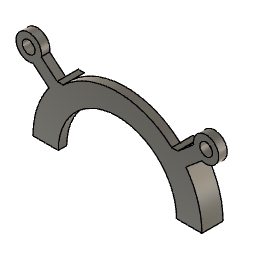
v2 - Timer - Assembly (Autodesk Fusion 360 archive; units mm, degrees)
design "v2 - Timer - Led ring insert"
Autodesk Fusion 360 part; units mm, degrees
note: some values were not read from the file. Chosen so that the rebuilt part matches the saved one: which bodies a step acts on; which face or edge a step refers to. Set by a fixed rule: which sketch regions a step uses.
sketch "Sketch1" plane through (0, 0, 0) normal (0, 1, 0) x (1, 0, 0)
  line L0 (0, 0) -> (50, 0)
  line L1 (50, 0) -> (50, -38.7)
  line L2 (50, -38.7) -> (0, -38.7)
  line L3 (0, -38.7) -> (0, 0)
  line L4 (0, -38.7) -> (50, -38.7)
  line L5 (50, -38.7) -> (50, -23.7)
  line L6 (50, -23.7) -> (0, -23.7)
  line L7 (0, -23.7) -> (0, -38.7)
  circle A0 centre (46, -17.7) radius 1.5
  circle A1 centre (4, -17.7) radius 1.5
  circle A2 centre (25, 0) radius 20
  circle A3 centre (25, 0) radius 1.5
  line L8 (3.0333, -16.5531) -> (24.0333, 1.1469)
  line L9 (4.9667, -18.8469) -> (25.9667, -1.1469)
  line L10 (45.0333, -18.8469) -> (24.0333, -1.1469)
  line L11 (46.9667, -16.5531) -> (25.9667, 1.1469)
  circle A4 centre (4, -17.7) radius 3
  circle A5 centre (46, -17.7) radius 3
  circle A6 centre (25, 0) radius 14
  circle A7 centre (25, 0) radius 19
  line L12 (39.2828, -14.0001) -> (10.7172, -14.0001)
  dimension "d1" = 50
  dimension "d2" = 38.7
  dimension "d3" = 15
  dimension "d4" = 3
  dimension "d5" = 3
  dimension "d6" = 21
  dimension "d7" = 4
  dimension "d8" = 21
  dimension "d9" = 4
  dimension "d16" = 3
  dimension "d17" = 6
  dimension "d18" = 6
  dimension "d22" = 28
  dimension "d40" = 40
  dimension "d41" = 38
  constraint horizontal L0
  constraint vertical L1
  constraint horizontal L2
  constraint vertical L3
  constraint coincident L0.start L3.end
  constraint horizontal L4
  constraint vertical L5
  constraint horizontal L6
  constraint vertical L7
  constraint coincident A1 L8.start
  constraint coincident A3 L8.end
  constraint tangent A3 L8
  constraint coincident A1 L9.start
  constraint coincident A3 L9.end
  constraint tangent A3 L9
  constraint coincident A0 L10.start
  constraint coincident A3 L10.end
  constraint tangent A3 L10
  constraint coincident A0 L11.start
  constraint coincident A3 L11.end
  constraint tangent A3 L11
  constraint tangent A1 L8
  constraint tangent A1 L9
  constraint tangent A0 L10
  constraint tangent A0 L11
  constraint concentric A1 A4
  constraint concentric A0 A5
  constraint concentric A2 A6
  constraint concentric A6 A7
  constraint coincident A2 L12.start
  constraint coincident L10 L12.start
  constraint coincident A2 L12.end
  constraint coincident L9 L12.end
  constraint horizontal L12
  measures "d1" distance of L0.start L0.end
  measures "d2" distance of L0.start L2.end
  measures "d3" distance of L2.end L6.end
  measures "d4" diameter of A0
  measures "d5" diameter of A1
  measures "d6" distance of L2 A0.centre
  measures "d7" distance of L1 A0.centre
  measures "d8" distance of L2 A1.centre
  measures "d9" distance of L3 A1.centre
  measures "d16" diameter of A3
  measures "d17" diameter of A4
  measures "d18" diameter of A5
  measures "d22" diameter of A6
  measures "d40" diameter of A2
  measures "d41" diameter of A7
extrude "Extrude6" add sketch "Sketch1" along normal blind 2 contours L0 L11 A6 A7 | L0 A2 L11 A7 | L0 L8 A6 A7 | L10 L11 A6 A7 | L0 A2 L8 A7 | A2 L10 L11 A7 | L8 L9 A6 A7 | L10 A6 A7 L12 | A2 L10 L11 A5 | A2 L8 L9 A7 | L10 A7 L12 | L9 A6 A7 L12 | A7 L12 | A2 A7 L12 | A0 L10 L11 A5 | A0 L10 L11 A5 | L9 A7 L12 makes body 1
extrude "Extrude8" add sketch "Sketch1" along normal blind 2 contours A2 L8 L9 A7 | A2 L8 L9 A4 | A1 L8 L9 A4 | A1 L8 L9 A4 bodies 1
extrude "Extrude9" cut sketch "Sketch1" along normal blind 4 contours L0 A2 L11 A7 | L0 A2 L8 A7 | A2 L10 L11 A7 | A2 L8 L9 A7 | L10 A7 L12 | A2 A7 L12 | L9 A7 L12 bodies 1 makes body 2 at (7.1209, 0, 14.8513) makes body 3 at (8.0709, 0, 3.5062)
extrude "Extrude10" add sketch "Sketch1" along normal blind 5 contours L0 A2 L11 A7 | L0 A2 L8 A7 | A2 L10 L11 A7 | A2 L8 L9 A7 | L10 A7 L12 | A2 A7 L12 | L9 A7 L12 bodies 1 2 3
extrude "Extrude11" cut sketch "Sketch1" along normal blind 14 contours A2 A7 L12 bodies 1
